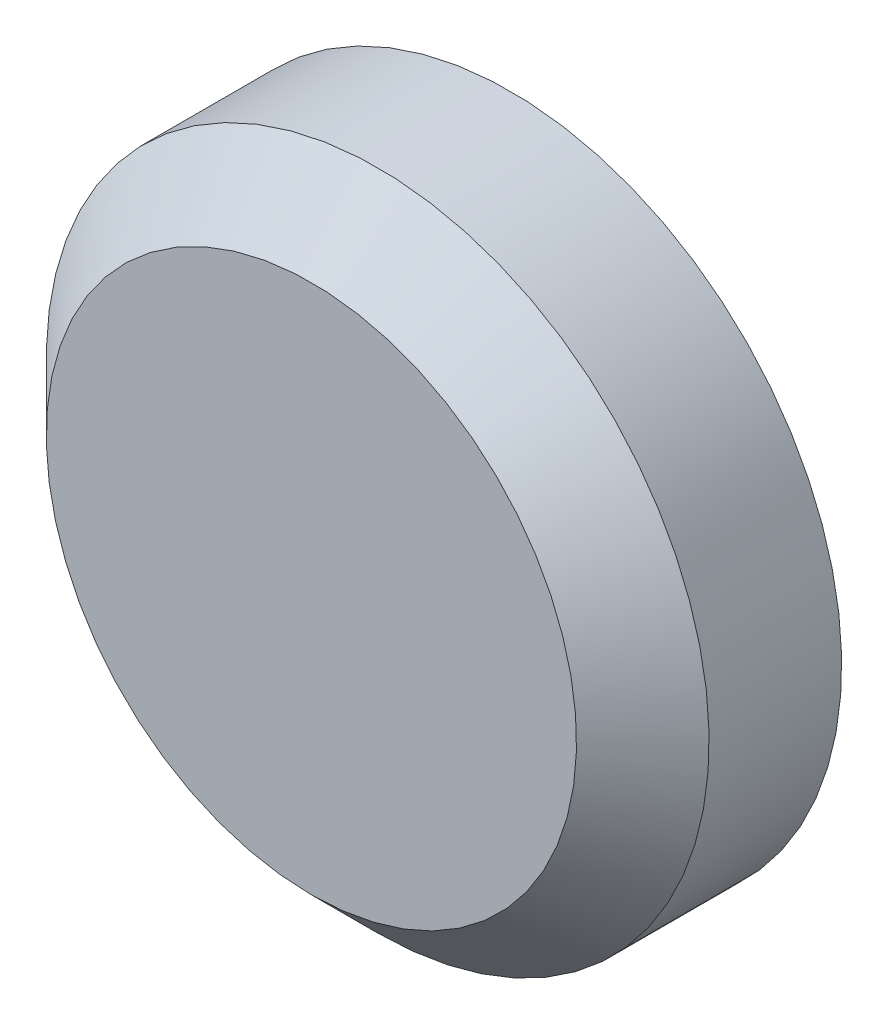
# Autodesk Inventor part: Dose_oben
Saved by Autodesk Inventor 2020 (Build 240168000, 168)
## iProperties
Created: 2020-03-21
Part Number: Dose_oben
Material: Generisch
Document SubType Name: Modeling
Designer: franz
Density: 1 g/cm^3
Appearance: Vorgabe
Author: franz
Autodesk Inventor part; units mm, degrees
ref_plane "YZ Plane" through (0, 0, 0) normal (1, 0, 0) x (0, 1, 0)
ref_plane "XZ Plane" through (0, 0, 0) normal (0, 1, 0) x (-1, 0, 0)
ref_plane "XY Plane" through (0, 0, 0) normal (0, 0, 1) x (1, 0, 0)
sketch "Skizze2" plane through (0, 0, 0) normal (1, 0, 0) x (0, 1, 0)
  line L0 (0, -14.6074) -> (0, 127.4912)
  line L1 (0, 0) -> (-50, 0)
  line L2 (-50, 0) -> (-50, 20)
  line L3 (-50, 20) -> (-40, 30)
  line L4 (-40, 30) -> (0, 30)
  dimension "d0" = 30
  dimension "d1" = 100
  dimension "d2" = 45
  dimension "d3" = 10
  constraints: 10 end point, 2 horizontal, 2 vertical, 1 perpendicular, 1 point on line
  measures "d0" distance between parallel lines of L1 L4
  measures "d1" diameter of L2 L0
  measures "d2" angle of L4 L3
  measures "d3" distance from line of L4 L2.end
revolve "Umdrehung1" add sketch "Skizze2" angle 360 about axis through (0, 0, -14.6074) along (0, 0, 1)
